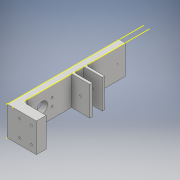
# Autodesk Inventor part: Подпора
Saved by Autodesk Inventor 2018 (Build 220112000, 112)
## iProperties
Created: 2023-02-19
Part Number: Подпора
Material: Типовые
Document SubType Name: Modeling
Designer: exper
Density: 1 g/cm^3
Appearance: По умолчанию
Author: exper
Autodesk Inventor part; units mm, degrees
ref_plane "YZ Plane" through (0, 0, 0) normal (1, 0, 0) x (0, 1, 0)
ref_plane "XZ Plane" through (0, 0, 0) normal (0, 1, 0) x (-1, 0, 0)
ref_plane "XY Plane" through (0, 0, 0) normal (0, 0, 1) x (1, 0, 0)
sketch "Эскиз1" plane through (0, 0, 0) normal (0, 1, 0) x (-1, 0, 0)
  line L0 (0, 0) -> (-60, 0)
  line L1 (-60, 0) -> (-60, -60)
  line L2 (-60, -60) -> (0, -60)
  line L3 (0, -60) -> (0, 0)
  dimension "d0" = 60
  dimension "d1" = 60
  constraints: 8 end point, 2 parallel, 1 horizontal, 1 perpendicular
  measures "d0" distance of L2.end L1.end
  measures "d1" distance of L1.end L0.end
extrude "Выдавливание1" add sketch "Эскиз1" along normal blind 20
sketch "Эскиз2" plane through (0, 20, 0) normal (0, 1, 0) x (1, 0, 0)
  line L0 (0, 0) -> (60, 0) projected
  line L1 (0, 0) -> (12, 0)
  line L2 (12, 0) -> (12, 60)
  line L3 (60, 60) -> (0, 60) projected
  line L4 (0, 60) -> (0, 0) projected
  line L5 (0, 60) -> (0, 0)
  dimension "d4" = 12
  constraints: 6 end point, 2 point on line, 1 collinear, 1 perpendicular
  measures "d4" distance of L0.start L1.end
extrude "Выдавливание2" add sketch "Эскиз2" along normal blind 260
sketch "Эскиз3" plane through (0, 20, 0) normal (0, 1, 0) x (1, 0, 0)
  point P0 (0, 0)
  point P1 (26, 13)
  point P2 (26, 47)
  point P3 (50.2241, 13)
  point P4 (50.2241, 47)
hole "Отверстие1" at (26, 20, -13) at (26, 20, -47) at (50.2241, 20, -13) at (50.2241, 20, -47) direction (0, -1, 0) diameter 4 depth 40 tip angle 118
sketch "Эскиз4" plane through (12, 20, 0) normal (1, 0, 0) x (0, 0, -1)
  point P0 (0, -20)
  point P1 (30, 88)
  dimension "d14" = 0
  constraints: 2 other
extrude "Выдавливание3" [suppressed]
sketch "Эскиз5" plane through (12, 20, 0) normal (1, 0, 0) x (0, 0, -1)
  point P0 (0, -20)
sketch "Эскиз6" plane through (0, 0, 0) normal (0, 0, 1) x (1, 0, 0)
  line L0 (0, 0) -> (0, 280) projected
  line L1 (12, 20) -> (12, 280) projected
sketch "Эскиз7" plane through (60, 0, -60) normal (0, 0, -1) x (-1, 0, 0)
  point P0 (60, 0)
sketch "Эскиз8" plane through (12, 20, 0) normal (1, 0, 0) x (0, 0, -1)
  circle A0 centre (30, 80) radius 11.5
  point P0 (0, -20)
  point P1 (0, 80)
  dimension "d17" = 23
  constraints: 1 centre point, 1 coincident
  measures "d17" diameter of A0
extrude "Выдавливание4" cut sketch "Эскиз8" against normal blind 100
sketch "Эскиз9" plane through (0, 0, -60) normal (-1, 0, 0) x (0, 0, 1)
  circle A0 centre (29.731, 99.8395) radius 12.5286
  point P0 (60, 0)
  point P1 (0, 80)
  constraints: 1 centre point
extrude "Выдавливание5" add sketch "Эскиз9" against normal blind 12
sketch "Эскиз10" plane through (0, 0, -60) normal (-1, 0, 0) x (0, 0, 1)
  line L0 (0, 0) -> (0, 280) projected
  circle A0 centre (30, 60) radius 11
  circle A1 centre (22, 80) radius 2
  circle A2 centre (38, 80) radius 2
  point P0 (60, 0)
  point P1 (0, 60)
  point P2 (0, 80)
  point P3 (30, 80)
  dimension "d22" = 22
  dimension "d23" = 4
  dimension "d24" = 4
  constraints: 3 centre point, 3 coincident, 1 point on line
  measures "d22" diameter of A0
  measures "d23" diameter of A1
  measures "d24" diameter of A2
extrude "Выдавливание6" cut sketch "Эскиз10" against normal blind 12
sketch "Эскиз11" plane through (0, 0, 0) normal (0, -1, 0) x (1, 0, 0)
  point P0 (0, 0)
fillet "Сопряжение1" radius 10 1 edges at (12, 20, -30)
sketch "Эскиз12" plane through (0, 0, -60) normal (-1, 0, 0) x (0, 0, 1)
  line L0 (0, 120) -> (60, 120)
  line L1 (60, 120) -> (60, 125)
  line L2 (60, 125) -> (0, 125)
  line L3 (0, 125) -> (0, 120)
  point P0 (60, 0)
  dimension "d28" = 60
  dimension "d29" = 5
  constraints: 8 end point, 2 parallel, 1 horizontal, 1 perpendicular
  measures "d28" distance of L2.end L1.end
  measures "d29" distance of L1.end L0.end
extrude "Выдавливание7" add sketch "Эскиз12" against normal blind 50
fillet "Сопряжение2" radius 5 1 edges at (12, 125, -30)
sketch "Эскиз13" plane through (50, 125, 0) normal (0, 1, 0) x (1, 0, 0)
  circle A0 centre (-19, 30) radius 2
  point P0 (-50, 0)
  dimension "d33" = 4
  constraints: 1 centre point, 1 coincident
  measures "d33" diameter of A0
extrude "Выдавливание8" cut sketch "Эскиз13" against normal blind 50
sketch "Эскиз14" plane through (0, 0, -60) normal (-1, 0, 0) x (0, 0, 1)
  line L0 (0, 0) -> (0, 280) projected
  line L1 (0, 145) -> (60, 145)
  line L2 (60, 145) -> (60, 150)
  line L3 (60, 150) -> (0, 150)
  line L4 (0, 150) -> (0, 145)
  point P0 (60, 0)
  dimension "d36" = 60
  dimension "d37" = 5
  constraints: 8 end point, 2 parallel, 1 horizontal, 1 perpendicular, 1 point on line
  measures "d36" distance of L3.end L2.end
  measures "d37" distance of L2.end L1.end
extrude "Выдавливание9" add sketch "Эскиз14" against normal blind 50
fillet "Сопряжение3" radius 5 1 edges at (12, 150, -30)
sketch "Эскиз15" plane through (12, 145, -60) normal (0, -1, 0) x (1, 0, 0)
  circle A0 centre (19, 30) radius 2 projected
  circle A1 centre (19, 30) radius 2
  circle A2 centre (19, 30) radius 2
  point P0 (-12, 60)
  point P1 (3.4297, 11.4015)
  dimension "d41" = 4
  constraints: 5 coincident, 2 centre point, 1 concentric
  measures "d41" diameter of A2
extrude "Выдавливание10" cut sketch "Эскиз15" against normal blind 50
sketch "Эскиз16" plane through (0, 0, -60) normal (-1, 0, 0) x (0, 0, 1)
  line L0 (0, 0) -> (0, 280) projected
  circle A0 centre (30, 215) radius 0.5
  point P0 (60, 0)
  point P1 (0, 215)
  point P2 (0, 215)
  dimension "d44" = 1
  constraints: 2 coincident, 1 centre point, 1 point on line
  measures "d44" diameter of A0
extrude "Выдавливание11" cut sketch "Эскиз16" against normal blind 100
sketch "Эскиз17" plane through (12, 280, 0) normal (1, 0, 0) x (0, 0, -1)
  point P0 (0, -280)
sketch "Эскиз18" plane through (12, 280, 0) normal (1, 0, 0) x (0, 0, -1)
  line L0 (0, -125) -> (0, 0) projected
  line L1 (60, -280) -> (60, 0) projected
  line L2 (0, -80) -> (0, -50)
  line L3 (0, -50) -> (5, -50)
  line L4 (5, -50) -> (5, -80)
  line L5 (5, -80) -> (0, -80)
  line L6 (0, -80) -> (0, -50)
  point P0 (0, -280)
  point P1 (30, -80)
  point P2 (30, -50)
  dimension "d47" = 5
  constraints: 10 end point, 2 parallel, 1 horizontal, 1 perpendicular, 1 point on line
  measures "d47" distance of L4.end L5.end
extrude "Выдавливание12" add sketch "Эскиз18" along normal blind 44.5
sketch "Эскиз19" plane through (0, 0, 0) normal (0, 0, 1) x (1, 0, 0)
  circle A0 centre (52.5, 223) radius 2
  circle A1 centre (52.5, 207) radius 2
  point P0 (0, 0)
  point P1 (52.5, 215)
  dimension "d50" = 4
  dimension "d51" = 4
  constraints: 2 centre point, 2 coincident
  measures "d50" diameter of A0
  measures "d51" diameter of A1
extrude "Выдавливание13" cut sketch "Эскиз19" against normal blind 45
fillet "Сопряжение4" radius 10 1 edges at (12, 215, -5)
sketch "Эскиз20" plane through (12, 280, 0) normal (1, 0, 0) x (0, 0, -1)
  line L0 (0, -280) -> (0, 0) projected
  line L1 (0, -50.033) -> (60, -50.033)
  line L2 (60, -280) -> (60, 0) projected
  line L3 (60, -50.033) -> (60, 0)
  line L4 (60, 0) -> (0, 0)
  line L5 (0, 0) -> (0, -50.033)
  constraints: 8 end point, 2 perpendicular, 1 collinear, 1 horizontal, 1 point on line
extrude "Выдавливание14" cut sketch "Эскиз20" against normal blind 100
sketch "Эскиз21" plane through (0, 0, 0) normal (0, 0, 1) x (1, 0, 0)
  line L0 (22, 230) -> (12, 230) projected
  line L1 (22, 200) -> (56.5, 200) projected
  line L2 (12, 230) -> (56.5, 230)
  line L3 (56.5, 230) -> (56.5, 200)
  line L4 (56.5, 200) -> (12, 200)
  line L5 (12, 200) -> (12, 230)
  point P0 (0, 0)
  constraints: 8 end point, 2 parallel, 1 horizontal, 1 perpendicular
extrude "Выдавливание15" cut sketch "Эскиз21" against normal blind 100
